Autodesk Fusion 360 part; units mm, degrees
(part 2 of 2)
sketch "Sketch22" plane through (30.25, 0, 0) normal (1, 0, 0) x (0, 1, 0)
  line L0 (-38.25, -13.3) -> (17.05, -13.3)
  line L1 (17.05, -13.3) -> (17.05, 8.2)
  line L2 (17.05, 8.2) -> (-38.25, 8.2)
  line L3 (-38.25, 8.2) -> (-38.25, -13.3)
  line L4 (-31.6678, 17.3589) -> (-31.6678, 16.8193)
  spline S0 degree 3 poles (-31.6678, 16.8193) (-33.0492, 16.7037) (-33.1985, 16.5882) (-33.1985, 14.5079) knots 0 0 0 0 1 1 1 1
  line L5 (-33.1985, 14.5079) -> (-33.1985, 10.4432)
  spline S1 degree 3 poles (-33.1985, 10.4432) (-33.1985, 7.3806) (-32.2277, 5.666) (-30.0251, 5.666) knots 0 0 0 0 1 1 1 1
  spline S2 degree 3 poles (-30.0251, 5.666) (-27.7665, 5.666) (-26.6466, 7.4384) (-26.6466, 10.8094) knots 0 0 0 0 1 1 1 1
  line L6 (-26.6466, 10.8094) -> (-26.6466, 11.9651)
  spline S3 degree 3 poles (-26.6466, 11.9651) (-26.6466, 14.1612) (-26.7399, 15.2398) (-26.8147, 15.8177) knots 0 0 0 0 1 1 1 1
  spline S4 degree 3 poles (-26.8147, 15.8177) (-26.9079, 16.5111) (-27.4306, 16.7423) (-28.6251, 16.8193) knots 0 0 0 0 1 1 1 1
  line L7 (-28.6251, 16.8193) -> (-28.6251, 17.3589)
  line L8 (-28.6251, 17.3589) -> (-24.0707, 17.3589)
  line L9 (-24.0707, 17.3589) -> (-24.0707, 16.8193)
  spline S5 degree 3 poles (-24.0707, 16.8193) (-25.0039, 16.7808) (-25.4893, 16.5111) (-25.5826, 15.8177) knots 0 0 0 0 1 1 1 1
  spline S6 degree 3 poles (-25.5826, 15.8177) (-25.6572, 15.2398) (-25.7506, 14.1612) (-25.7506, 11.9651) knots 0 0 0 0 1 1 1 1
  line L10 (-25.7506, 11.9651) -> (-25.7506, 10.5973)
  spline S7 degree 3 poles (-25.7506, 10.5973) (-25.7506, 8.7289) (-26.0866, 7.1302) (-27.1132, 5.9937) knots 0 0 0 0 1 1 1 1
  spline S8 degree 3 poles (-27.1132, 5.9937) (-27.9346, 5.0691) (-29.2598, 4.5488) (-30.5665, 4.5488) knots 0 0 0 0 1 1 1 1
  spline S9 degree 3 poles (-30.5665, 4.5488) (-31.7238, 4.5488) (-32.9558, 4.78) (-33.8892, 5.57) knots 0 0 0 0 1 1 1 1
  spline S10 degree 3 poles (-33.8892, 5.57) (-34.8784, 6.3982) (-35.2892, 7.7851) (-35.2892, 10.0582) knots 0 0 0 0 1 1 1 1
  line L11 (-35.2892, 10.0582) -> (-35.2892, 14.5079)
  spline S11 degree 3 poles (-35.2892, 14.5079) (-35.2892, 16.5882) (-35.4386, 16.7037) (-36.9319, 16.8193) knots 0 0 0 0 1 1 1 1
  line L12 (-36.9319, 16.8193) -> (-36.9319, 17.3589)
  line L13 (-36.9319, 17.3589) -> (-31.6678, 17.3589)
  spline S12 degree 3 poles (0.187, 14.4116) (-0.1926, 15.5288) (-0.8466, 16.8771) (-2.6182, 16.8771) knots 0 0 0 0 1 1 1 1
  spline S13 degree 3 poles (-2.6182, 16.8771) (-4.0105, 16.8771) (-4.7699, 15.9525) (-4.7699, 14.8546) knots 0 0 0 0 1 1 1 1
  spline S14 degree 3 poles (-4.7699, 14.8546) (-4.7699, 13.7757) (-3.9262, 13.063) (-2.3021, 12.3889) knots 0 0 0 0 1 1 1 1
  line L14 (-2.3021, 12.3889) -> (-1.7535, 12.1577)
  spline S15 degree 3 poles (-1.7535, 12.1577) (-0.1083, 11.4836) (1.4104, 10.4625) (1.4104, 8.4595) knots 0 0 0 0 1 1 1 1
  spline S16 degree 3 poles (1.4104, 8.4595) (1.4104, 6.1668) (-0.5513, 4.5489) (-3.3989, 4.5489) knots 0 0 0 0 1 1 1 1
  spline S17 degree 3 poles (-3.3989, 4.5489) (-4.2004, 4.5489) (-4.9598, 4.7029) (-5.5082, 4.8763) knots 0 0 0 0 1 1 1 1
  spline S18 degree 3 poles (-5.5082, 4.8763) (-6.0987, 5.0497) (-6.4783, 5.2038) (-6.7317, 5.2808) knots 0 0 0 0 1 1 1 1
  spline S19 degree 3 poles (-6.7317, 5.2808) (-6.9002, 5.7818) (-7.1534, 7.0914) (-7.3646, 8.2666) knots 0 0 0 0 1 1 1 1
  line L15 (-7.3646, 8.2666) -> (-6.7317, 8.4595)
  spline S20 degree 3 poles (-6.7317, 8.4595) (-6.3097, 7.4576) (-5.1705, 5.3193) (-2.9983, 5.3193) knots 0 0 0 0 1 1 1 1
  spline S21 degree 3 poles (-2.9983, 5.3193) (-1.627, 5.3193) (-0.7836, 6.3017) (-0.7836, 7.4964) knots 0 0 0 0 1 1 1 1
  spline S22 degree 3 poles (-0.7836, 7.4964) (-0.7836, 8.5748) (-1.3528, 9.3455) (-3.0191, 10.0967) knots 0 0 0 0 1 1 1 1
  line L16 (-3.0191, 10.0967) -> (-3.6939, 10.4049)
  spline S23 degree 3 poles (-3.6939, 10.4049) (-5.0865, 11.0598) (-6.8581, 12.0807) (-6.8581, 13.9686) knots 0 0 0 0 1 1 1 1
  spline S24 degree 3 poles (-6.8581, 13.9686) (-6.8581, 15.9911) (-5.1918, 17.6476) (-2.3653, 17.6476) knots 0 0 0 0 1 1 1 1
  spline S25 degree 3 poles (-2.3653, 17.6476) (-1.7959, 17.6476) (-1.0365, 17.5708) (-0.4457, 17.3781) knots 0 0 0 0 1 1 1 1
  spline S26 degree 3 poles (-0.4457, 17.3781) (-0.1083, 17.2623) (0.187, 17.2238) (0.4401, 17.1275) knots 0 0 0 0 1 1 1 1
  spline S27 degree 3 poles (0.4401, 17.1275) (0.5244, 16.4533) (0.6508, 15.6058) (0.862, 14.5269) knots 0 0 0 0 1 1 1 1
  line L17 (0.862, 14.5269) -> (0.187, 14.4116)
  spline S28 degree 3 poles (-11.6262, 14.0263) (-12.2235, 16.2222) (-13.3996, 16.8771) (-15.1357, 16.8771) knots 0 0 0 0 1 1 1 1
  spline S29 degree 3 poles (-15.1357, 16.8771) (-18.197, 16.8771) (-19.5782, 14.2382) (-19.5782, 11.387) knots 0 0 0 0 1 1 1 1
  spline S30 degree 3 poles (-19.5782, 11.387) (-19.5782, 7.8043) (-17.8609, 5.3193) (-15.1357, 5.3193) knots 0 0 0 0 1 1 1 1
  spline S31 degree 3 poles (-15.1357, 5.3193) (-13.1196, 5.3193) (-12.1864, 6.3982) (-11.2156, 8.44) knots 0 0 0 0 1 1 1 1
  line L18 (-11.2156, 8.44) -> (-10.693, 8.3244)
  spline S32 degree 3 poles (-10.693, 8.3244) (-10.9169, 7.3998) (-11.3278, 5.8587) (-11.6262, 5.1267) knots 0 0 0 0 1 1 1 1
  spline S33 degree 3 poles (-11.6262, 5.1267) (-12.149, 4.9728) (-13.8288, 4.5489) (-15.1357, 4.5489) knots 0 0 0 0 1 1 1 1
  spline S34 degree 3 poles (-15.1357, 4.5489) (-20.0262, 4.5489) (-22.0047, 7.8428) (-22.0047, 10.8864) knots 0 0 0 0 1 1 1 1
  spline S35 degree 3 poles (-22.0047, 10.8864) (-22.0047, 14.9317) (-18.9808, 17.6476) (-14.7996, 17.6476) knots 0 0 0 0 1 1 1 1
  spline S36 degree 3 poles (-14.7996, 17.6476) (-13.1943, 17.6476) (-11.9623, 17.2623) (-11.4397, 17.1468) knots 0 0 0 0 1 1 1 1
  spline S37 degree 3 poles (-11.4397, 17.1468) (-11.2904, 16.0681) (-11.2156, 15.2206) (-11.1039, 14.1032) knots 0 0 0 0 1 1 1 1
  line L19 (-11.1039, 14.1032) -> (-11.6262, 14.0263)
  line L20 (8.2475, 11.1946) -> (8.2475, 7.7658)
  spline S38 degree 3 poles (8.2475, 7.7658) (8.2475, 5.9552) (8.494, 5.57) (9.8081, 5.6082) knots 0 0 0 0 1 1 1 1
  spline S39 degree 3 poles (9.8081, 5.6082) (11.1633, 5.6082) (12.5594, 6.3209) (12.5594, 8.3051) knots 0 0 0 0 1 1 1 1
  spline S40 degree 3 poles (12.5594, 8.3051) (12.5594, 10.2701) (11.04, 11.1946) (8.9457, 11.1946) knots 0 0 0 0 1 1 1 1
  line L21 (8.9457, 11.1946) -> (8.2475, 11.1946)
  line L22 (8.2475, 11.8881) -> (9.0689, 11.8881)
  spline S41 degree 3 poles (9.0689, 11.8881) (10.8347, 11.8881) (11.9435, 12.6585) (11.9435, 14.2765) knots 0 0 0 0 1 1 1 1
  spline S42 degree 3 poles (11.9435, 14.2765) (11.9435, 16.0488) (10.6088, 16.6267) (9.3565, 16.6267) knots 0 0 0 0 1 1 1 1
  spline S43 degree 3 poles (9.3565, 16.6267) (8.8224, 16.6267) (8.535, 16.5882) (8.4118, 16.5304) knots 0 0 0 0 1 1 1 1
  spline S44 degree 3 poles (8.4118, 16.5304) (8.2475, 16.4533) (8.2475, 16.1259) (8.2475, 15.6636) knots 0 0 0 0 1 1 1 1
  line L23 (8.2475, 15.6636) -> (8.2475, 11.8881)
  spline S45 degree 3 poles (10.0134, 17.3589) (11.6149, 17.3589) (12.4361, 17.166) (13.1756, 16.723) knots 0 0 0 0 1 1 1 1
  spline S46 degree 3 poles (13.1756, 16.723) (13.9145, 16.2607) (14.3251, 15.548) (14.3251, 14.5269) knots 0 0 0 0 1 1 1 1
  spline S47 degree 3 poles (14.3251, 14.5269) (14.3251, 12.8704) (12.621, 11.9844) (11.4096, 11.7727) knots 0 0 0 0 1 1 1 1
  line L24 (11.4096, 11.7727) -> (11.4096, 11.734)
  spline S48 degree 3 poles (11.4096, 11.734) (13.5039, 11.5028) (15.1056, 10.4432) (15.1056, 8.517) knots 0 0 0 0 1 1 1 1
  spline S49 degree 3 poles (15.1056, 8.517) (15.1056, 7.1492) (14.387, 6.2441) (13.2576, 5.6082) knots 0 0 0 0 1 1 1 1
  spline S50 degree 3 poles (13.2576, 5.6082) (12.2925, 5.0691) (10.8347, 4.8378) (9.3359, 4.8378) knots 0 0 0 0 1 1 1 1
  line L25 (9.3359, 4.8378) -> (4.2231, 4.8378)
  line L26 (4.2231, 4.8378) -> (4.2231, 5.3771)
  spline S51 degree 3 poles (4.2231, 5.3771) (5.8248, 5.4929) (5.9889, 5.6468) (5.9889, 7.7273) knots 0 0 0 0 1 1 1 1
  line L27 (5.9889, 7.7273) -> (5.9889, 14.4694)
  spline S52 degree 3 poles (5.9889, 14.4694) (5.9889, 16.5496) (5.8248, 16.7037) (4.3464, 16.8193) knots 0 0 0 0 1 1 1 1
  line L28 (4.3464, 16.8193) -> (4.3464, 17.3589)
  line L29 (4.3464, 17.3589) -> (10.0134, 17.3589)
  spline S53 degree 3 poles (-4.0937, 0.2766) (-8.1951, 3.9023) (-19.0499, 1.7495) (-23.1742, 0.0729) knots 0 0 0 0 1 1 1 1
  spline S54 degree 3 poles (-23.1742, 0.0729) (-28.8848, -2.1028) (-34.2101, -5.1847) (-38.0625, -2.7144) knots 0 0 0 0 1 1 1 1
  spline S55 degree 2 poles (-38.0625, -2.7144) (-38.0852, -2.6918) (-38.1305, -2.6918) knots 0 0 0 1 1 1
  spline S56 degree 3 poles (-38.1305, -2.6918) (-38.1305, -2.7144) (-38.1305, -2.7598) (-38.1078, -2.7827) knots 0 0 0 0 1 1 1 1
  spline S57 degree 3 poles (-38.1078, -2.7827) (-33.8476, -6.3858) (-23.2196, -4.414) (-19.1406, -2.6694) knots 0 0 0 0 1 1 1 1
  spline S58 degree 3 poles (-19.1406, -2.6694) (-13.4073, -0.4712) (-7.9461, 2.656) (-4.139, 0.1862) knots 0 0 0 0 1 1 1 1
  spline S59 degree 3 poles (-4.139, 0.1862) (-4.1161, 0.1862) (-4.071, 0.1862) (-4.071, 0.2086) knots 0 0 0 0 1 1 1 1
  spline S60 degree 2 poles (-4.071, 0.2086) (-4.071, 0.2315) (-4.0937, 0.2766) knots 0 0 0 1 1 1
  spline S61 degree 3 poles (-4.0937, 0.2766) (-8.1951, 3.9023) (-19.0499, 1.7495) (-23.1742, 0.0729) knots 0 0 0 0 1 1 1 1
  spline S62 degree 3 poles (-23.1742, 0.0729) (-28.8848, -2.1028) (-34.2101, -5.1847) (-38.0625, -2.7144) knots 0 0 0 0 1 1 1 1
  spline S63 degree 2 poles (-38.0625, -2.7144) (-38.0852, -2.6918) (-38.1305, -2.6918) knots 0 0 0 1 1 1
  spline S64 degree 3 poles (-38.1305, -2.6918) (-38.1305, -2.7144) (-38.1305, -2.7598) (-38.1078, -2.7827) knots 0 0 0 0 1 1 1 1
  spline S65 degree 3 poles (-38.1078, -2.7827) (-33.8476, -6.3858) (-23.2196, -4.414) (-19.1406, -2.6694) knots 0 0 0 0 1 1 1 1
  spline S66 degree 3 poles (-19.1406, -2.6694) (-13.4073, -0.4712) (-7.9461, 2.656) (-4.139, 0.1862) knots 0 0 0 0 1 1 1 1
  spline S67 degree 3 poles (-4.139, 0.1862) (-4.1161, 0.1862) (-4.071, 0.1862) (-4.071, 0.2086) knots 0 0 0 0 1 1 1 1
  spline S68 degree 2 poles (-4.071, 0.2086) (-4.071, 0.2315) (-4.0937, 0.2766) knots 0 0 0 1 1 1
  spline S69 degree 3 poles (16.7317, 0.2766) (12.6752, 3.9023) (1.8206, 1.7495) (-2.3264, 0.0729) knots 0 0 0 0 1 1 1 1
  spline S70 degree 3 poles (-2.3264, 0.0729) (-8.0143, -2.1028) (-13.3396, -5.1847) (-17.192, -2.7144) knots 0 0 0 0 1 1 1 1
  spline S71 degree 3 poles (-17.192, -2.7144) (-17.2146, -2.6918) (-17.2599, -2.6918) (-17.2826, -2.6918) knots 0 0 0 0 1 1 1 1
  spline S72 degree 3 poles (-17.2826, -2.6918) (-17.2826, -2.7144) (-17.2826, -2.7598) (-17.2373, -2.7827) knots 0 0 0 0 1 1 1 1
  spline S73 degree 3 poles (-17.2373, -2.7827) (-12.977, -6.3858) (-2.3717, -4.414) (1.7073, -2.6694) knots 0 0 0 0 1 1 1 1
  spline S74 degree 3 poles (1.7073, -2.6694) (7.4407, -0.4712) (12.9018, 2.656) (16.7089, 0.1862) knots 0 0 0 0 1 1 1 1
  spline S75 degree 3 poles (16.7089, 0.1862) (16.7317, 0.1862) (16.7768, 0.1862) (16.7768, 0.2086) knots 0 0 0 0 1 1 1 1
  spline S76 degree 2 poles (16.7768, 0.2086) (16.7768, 0.2315) (16.7317, 0.2766) knots 0 0 0 1 1 1
  spline S77 degree 3 poles (16.7317, 0.2766) (12.6752, 3.9023) (1.8206, 1.7495) (-2.3264, 0.0729) knots 0 0 0 0 1 1 1 1
  spline S78 degree 3 poles (-2.3264, 0.0729) (-8.0143, -2.1028) (-13.3396, -5.1847) (-17.192, -2.7144) knots 0 0 0 0 1 1 1 1
  spline S79 degree 3 poles (-17.192, -2.7144) (-17.2146, -2.6918) (-17.2599, -2.6918) (-17.2826, -2.6918) knots 0 0 0 0 1 1 1 1
  spline S80 degree 3 poles (-17.2826, -2.6918) (-17.2826, -2.7144) (-17.2826, -2.7598) (-17.2373, -2.7827) knots 0 0 0 0 1 1 1 1
  spline S81 degree 3 poles (-17.2373, -2.7827) (-12.977, -6.3858) (-2.3717, -4.414) (1.7073, -2.6694) knots 0 0 0 0 1 1 1 1
  spline S82 degree 3 poles (1.7073, -2.6694) (7.4407, -0.4712) (12.9018, 2.656) (16.7089, 0.1862) knots 0 0 0 0 1 1 1 1
  spline S83 degree 3 poles (16.7089, 0.1862) (16.7317, 0.1862) (16.7768, 0.1862) (16.7768, 0.2086) knots 0 0 0 0 1 1 1 1
  spline S84 degree 2 poles (16.7768, 0.2086) (16.7768, 0.2315) (16.7317, 0.2766) knots 0 0 0 1 1 1
extrude "Extrude30" cut sketch "Sketch22" against normal blind 0.3 contours S53 S54 S55 S56 S57 S58 S59 S60 S61 S62 S63 S64 S65 S66 S67 S68 | S69 S70 S71 S72 S73 S74 S75 S76 S77 S78 S79 S80 S81 S82 S83 S84 bodies 2
extrude "Extrude31" cut sketch "Sketch22" along normal blind 0.3 from surface at -60.5 contours S53 S54 S55 S56 S57 S58 S59 S60 S61 S62 S63 S64 S65 S66 S67 S68 | S69 S70 S71 S72 S73 S74 S75 S76 S77 S78 S79 S80 S81 S82 S83 S84 bodies 2
equation "M4Insert = 5.45 mm"
equation "M4Spacing = 14 mm"
equation "PerfWidth = 65 mm"
equation "PerfHeigth = 45 mm"
equation "M3Insert = 4 mm"
equation "d15 = PerfHeigth"
equation "d16 = PerfWidth"
equation "d18 = M3Diameter"
equation "M3Diameter = 3.2 mm"
equation "PostDiameter = 4.2 mm"
equation "d93 = M3Insert"
equation "d135 = M4Spacing"
equation "d136 = M4Insert"
equation "d139 = PostDiameter"
